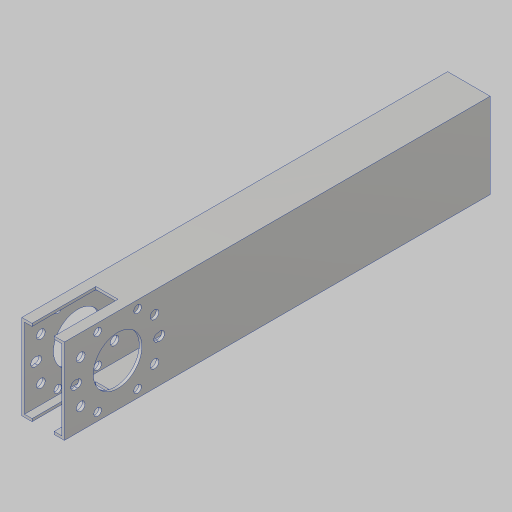
# Autodesk Inventor part: CL4-001
Saved by Autodesk Inventor 2023.5 (Build 275446000, 446)
## iProperties
RuleStatus: InUse
Created: 2025-02-03
Part Number: CL4-001
Material: Aluminum 6061
Document SubType Name: Modeling
Designer: brand
Mass: 304.185 g
Surface Area: 718.547 cm^2
Volume: 112.661 cm^3
Density: 2.7 g/cm^3
Appearance: Aluminum - Flat
AfterDocNew0: SHOW
AfterDocOpen0: SHOW
Author: brand
Autodesk Inventor part; units mm, degrees
ref_plane "YZ Plane" through (0, 0, 0) normal (1, 0, 0) x (0, 1, 0)
ref_plane "XZ Plane" through (0, 0, 0) normal (0, 1, 0) x (-1, 0, 0)
ref_plane "XY Plane" through (0, 0, 0) normal (0, 0, 1) x (1, 0, 0)
sketch "Sketch1" plane through (0, 0, 0) normal (0, 0, 1) x (1, 0, 0)
  line L0 (-12.7, -25.4) -> (12.7, -25.4)
  line L1 (12.7, -25.4) -> (12.7, 25.4)
  line L2 (12.7, 25.4) -> (-12.7, 25.4)
  line L3 (-12.7, 25.4) -> (-12.7, -25.4)
  line L4 (-12.7, -25.4) -> (12.7, 25.4) construction
  line L5 (12.7, -25.4) -> (-12.7, 25.4) construction
  line L6 (-11.1125, 23.8125) -> (11.1125, 23.8125)
  line L7 (11.1125, 23.8125) -> (11.1125, -23.8125)
  line L8 (11.1125, -23.8125) -> (-11.1125, -23.8125)
  line L9 (-11.1125, -23.8125) -> (-11.1125, 23.8125)
  point P0 (0, 0)
  dimension "width" = 25.4
  dimension "height" = 50.8
  dimension "thickness" = 1.5875
  constraints: 20 end point, 4 parallel, 2 midpoint, 2 perpendicular, 1 horizontal, 3 other
  measures "width" distance of L2.end L1.end
  measures "height" distance of L1.end L0.end
  measures "thickness" distance between parallel lines of L2 L6
extrude "Extrusion1" add sketch "Sketch1" along normal mid plane 254
sketch "Sketch2" plane through (12.7, -25.4, 127) normal (1, 0, 0) x (0, 0, -1)
  line L0 (254, 50.8) -> (254, 0) construction
  line L1 (254, 0) -> (0, 0) construction
  line L2 (0, 0) -> (0, 50.8) construction
  line L3 (0, 50.8) -> (254, 50.8) construction
  circle A0 centre (31.75, 25.4) radius 23.8125 construction
  circle A1 centre (31.75, 25.4) radius 25.4 construction
  point P0 (127, 25.4)
  point P1 (57.15, 25.4)
  point P2 (53.747, 38.1)
  point P3 (44.45, 47.397)
  point P4 (31.75, 50.8)
  point P5 (19.05, 47.397)
  point P6 (9.753, 38.1)
  point P7 (6.35, 25.4)
  point P8 (9.753, 12.7)
  point P9 (19.05, 3.403)
  point P10 (31.75, 0)
  point P11 (44.45, 3.403)
  point P12 (53.747, 12.7)
  point P13 (55.5625, 25.4)
  point P14 (43.6562, 46.0222)
  point P15 (19.8437, 46.0222)
  point P16 (7.9375, 25.4)
  point P17 (19.8437, 4.7778)
  point P18 (43.6562, 4.7778)
  dimension "d13" = 47.625
  dimension "d14" = 50.8
  dimension "d5" = 31.75
  dimension "d17" = 360
  dimension "d21" = 360
  constraints: 5 horizontal alignment, 2 coincident, 24 other
  measures "d5" distance from line of point (31.75, 25.4) L2
hole "Hole1" at (12.7, 0, 95.25) direction (-1, 0, 0) diameter 28.956 end through all
hole "Hole2" at (12.7, 12.7, 73.253) at (12.7, 0, 69.85) at (12.7, -12.7, 73.253) at (12.7, -12.7, 117.247) at (12.7, 0, 120.65) at (12.7, 12.7, 117.247) direction (-1, 0, 0) diameter 5.1054 end through all clearance for "Flat Head Machine Screw (82)" size "#10" standard "Ansi Unified Screw Threads"
hole "Hole3" at (12.7, -20.6222, 107.1562) at (12.7, -20.6222, 83.3438) at (12.7, 0, 119.0625) at (12.7, 20.6222, 107.1562) at (12.7, 20.6222, 83.3438) at (12.7, 0, 71.4375) direction (-1, 0, 0) diameter 4.4958 end through all clearance for "Flat Head Machine Screw (82)" size "#8" standard "Ansi Unified Screw Threads"
sketch "Sketch3" plane through (-12.7, 25.4, 127) normal (0, 1, 0) x (1, 0, 0)
  line L0 (0, 0) -> (25.4, 0) construction
  line L1 (6.096, 0) -> (19.304, 0)
  line L2 (19.304, 0) -> (19.304, 38.1)
  line L3 (19.304, 38.1) -> (6.096, 38.1)
  line L4 (6.096, 38.1) -> (6.096, 0)
  line L5 (25.4, 0) -> (0, 0) construction
  point P0 (12.7, 127)
  point P1 (12.7, 38.1)
  point P2 (12.7, 0)
  dimension "d37" = 13.208
  dimension "d38" = 38.1
  constraints: 8 end point, 2 midpoint, 2 parallel, 1 horizontal, 1 perpendicular, 1 point on line, 1 vertical alignment
  measures "d37" distance of L2.end L3.end
  measures "d38" distance of L3.end L1.start
extrude "Extrusion2" cut sketch "Sketch3" against normal through all
body "Solid1"
